Autodesk Fusion 360 part; units mm, degrees
(part 14 of 15)
  spline S147 degree 5 poles (-30.1889, -115.7087) (-30.196, -115.7166) (-30.2152, -115.7376) (-30.2465, -115.7718) (-30.29, -115.819) (-30.3459, -115.8792) (-30.4072, -115.9446) (-30.4688, -116.0097) (-30.5308, -116.0746) (-30.593, -116.1393) (-30.6557, -116.2038) (-30.7186, -116.268) (-30.7819, -116.332) (-30.8455, -116.3958) (-30.9093, -116.4594) (-30.9736, -116.5228) (-31.0381, -116.5859) (-31.1029, -116.6489) (-31.168, -116.7116) (-31.2334, -116.7741) (-31.2991, -116.8364) (-31.365, -116.8985) (-31.4313, -116.9604) (-31.4979, -117.0221) (-31.5647, -117.0836) (-31.6318, -117.1449) (-31.6992, -117.206) (-31.7668, -117.2669) (-31.8347, -117.3276) (-31.9029, -117.3881) (-31.9713, -117.4484) (-32.04, -117.5086) (-32.109, -117.5685) (-32.1782, -117.6282) (-32.2477, -117.6877) (-32.3174, -117.7471) (-32.3874, -117.8062) (-32.4576, -117.8652) (-32.5281, -117.9239) (-32.5988, -117.9825) (-32.6697, -118.0409) (-32.7409, -118.0991) (-32.8124, -118.1571) (-32.8697, -118.2034) (-32.9128, -118.238) (-32.9416, -118.261) (-32.956, -118.2725) knots 0.405839 0.405839 0.405839 0.405839 0.405839 0.405839 0.414286 0.428571 0.442857 0.457143 0.471429 0.485714 0.5 0.514286 0.528571 0.542857 0.557143 0.571429 0.585714 0.6 0.614286 0.628571 0.642857 0.657143 0.671429 0.685714 0.7 0.714286 0.728571 0.742857 0.757143 0.771429 0.785714 0.8 0.814286 0.828571 0.842857 0.857143 0.871429 0.885714 0.9 0.914286 0.928571 0.942857 0.957143 0.971429 0.985714 1 1 1 1 1 1
  arc A147 (-34.117, -117.6386) -> (-32.956, -118.2725) centre (2.0032, -52.8695) ccw
  spline S148 degree 5 poles (-34.117, -117.6386) (-34.1151, -117.6203) (-34.1113, -117.5836) (-34.1054, -117.5286) (-34.0975, -117.4554) (-34.0873, -117.3639) (-34.0769, -117.2726) (-34.0661, -117.1813) (-34.0551, -117.0901) (-34.0437, -116.9991) (-34.0321, -116.9081) (-34.0202, -116.8173) (-34.0079, -116.7266) (-33.9954, -116.6359) (-33.9826, -116.5454) (-33.9695, -116.455) (-33.956, -116.3647) (-33.9423, -116.2745) (-33.9283, -116.1845) (-33.9139, -116.0945) (-33.8993, -116.0047) (-33.8843, -115.915) (-33.869, -115.8254) (-33.8534, -115.7359) (-33.8375, -115.6466) (-33.8212, -115.5574) (-33.8046, -115.4683) (-33.7877, -115.3793) (-33.7705, -115.2905) (-33.7529, -115.2018) (-33.735, -115.1133) (-33.7168, -115.0249) (-33.6982, -114.9366) (-33.6792, -114.8485) (-33.6599, -114.7605) (-33.6403, -114.6727) (-33.6203, -114.585) (-33.5999, -114.4975) (-33.5792, -114.4101) (-33.5581, -114.3229) (-33.5366, -114.2358) (-33.5147, -114.149) (-33.4943, -114.0693) (-33.4781, -114.0072) (-33.4662, -113.9624) (-33.4589, -113.9349) (-33.4562, -113.9247) knots -1 -1 -1 -1 -1 -1 -0.985714 -0.971429 -0.957143 -0.942857 -0.928571 -0.914286 -0.9 -0.885714 -0.871429 -0.857143 -0.842857 -0.828571 -0.814286 -0.8 -0.785714 -0.771429 -0.757143 -0.742857 -0.728571 -0.714286 -0.7 -0.685714 -0.671429 -0.657143 -0.642857 -0.628571 -0.614286 -0.6 -0.585714 -0.571429 -0.557143 -0.542857 -0.528571 -0.514286 -0.5 -0.485714 -0.471429 -0.457143 -0.442857 -0.428571 -0.414286 -0.405839 -0.405839 -0.405839 -0.405839 -0.405839 -0.405839
  arc A148 (-34.5898, -113.2521) -> (-33.4562, -113.9247) centre (2.0032, -52.8695) ccw
  spline S149 degree 5 poles (-34.5898, -113.2521) (-34.5974, -113.2594) (-34.618, -113.279) (-34.6517, -113.3108) (-34.6985, -113.3549) (-34.7586, -113.4109) (-34.8243, -113.4718) (-34.8904, -113.5323) (-34.9569, -113.5927) (-35.0236, -113.6527) (-35.0907, -113.7126) (-35.158, -113.7721) (-35.2257, -113.8315) (-35.2937, -113.8906) (-35.3619, -113.9494) (-35.4305, -114.008) (-35.4994, -114.0664) (-35.5685, -114.1246) (-35.6379, -114.1825) (-35.7076, -114.2402) (-35.7776, -114.2977) (-35.8478, -114.3549) (-35.9183, -114.412) (-35.9891, -114.4687) (-36.0601, -114.5253) (-36.1314, -114.5817) (-36.203, -114.6378) (-36.2748, -114.6937) (-36.3469, -114.7494) (-36.4192, -114.8049) (-36.4918, -114.8602) (-36.5646, -114.9152) (-36.6377, -114.9701) (-36.711, -115.0247) (-36.7845, -115.0791) (-36.8583, -115.1334) (-36.9323, -115.1874) (-37.0065, -115.2412) (-37.081, -115.2947) (-37.1557, -115.3481) (-37.2307, -115.4013) (-37.3058, -115.4543) (-37.3812, -115.5071) (-37.4417, -115.5491) (-37.4872, -115.5806) (-37.5175, -115.6015) (-37.5327, -115.6119) knots 0.405839 0.405839 0.405839 0.405839 0.405839 0.405839 0.414286 0.428571 0.442857 0.457143 0.471429 0.485714 0.5 0.514286 0.528571 0.542857 0.557143 0.571429 0.585714 0.6 0.614286 0.628571 0.642857 0.657143 0.671429 0.685714 0.7 0.714286 0.728571 0.742857 0.757143 0.771429 0.785714 0.8 0.814286 0.828571 0.842857 0.857143 0.871429 0.885714 0.9 0.914286 0.928571 0.942857 0.957143 0.971429 0.985714 1 1 1 1 1 1
  arc A149 (-38.6455, -114.8968) -> (-37.5327, -115.6119) centre (2.0032, -52.8695) ccw
  spline S150 degree 5 poles (-38.6455, -114.8968) (-38.6423, -114.8786) (-38.6359, -114.8423) (-38.6262, -114.7879) (-38.613, -114.7154) (-38.5964, -114.6249) (-38.5794, -114.5345) (-38.5622, -114.4443) (-38.5446, -114.3541) (-38.5268, -114.2641) (-38.5087, -114.1742) (-38.4904, -114.0845) (-38.4717, -113.9949) (-38.4527, -113.9054) (-38.4335, -113.816) (-38.414, -113.7267) (-38.3941, -113.6376) (-38.374, -113.5487) (-38.3536, -113.4598) (-38.3328, -113.3711) (-38.3118, -113.2826) (-38.2905, -113.1942) (-38.2688, -113.1059) (-38.2469, -113.0178) (-38.2246, -112.9298) (-38.202, -112.842) (-38.1791, -112.7543) (-38.1559, -112.6668) (-38.1324, -112.5794) (-38.1086, -112.4922) (-38.0844, -112.4051) (-38.0599, -112.3183) (-38.035, -112.2316) (-38.0098, -112.145) (-37.9843, -112.0586) (-37.9584, -111.9724) (-37.9322, -111.8864) (-37.9057, -111.8005) (-37.8788, -111.7149) (-37.8515, -111.6294) (-37.8238, -111.5441) (-37.7958, -111.459) (-37.7698, -111.381) (-37.7492, -111.3202) (-37.7342, -111.2763) (-37.7249, -111.2494) (-37.7214, -111.2395) knots -1 -1 -1 -1 -1 -1 -0.985714 -0.971429 -0.957143 -0.942857 -0.928571 -0.914286 -0.9 -0.885714 -0.871429 -0.857143 -0.842857 -0.828571 -0.814286 -0.8 -0.785714 -0.771429 -0.757143 -0.742857 -0.728571 -0.714286 -0.7 -0.685714 -0.671429 -0.657143 -0.642857 -0.628571 -0.614286 -0.6 -0.585714 -0.571429 -0.557143 -0.542857 -0.528571 -0.514286 -0.5 -0.485714 -0.471429 -0.457143 -0.442857 -0.428571 -0.414286 -0.405839 -0.405839 -0.405839 -0.405839 -0.405839 -0.405839
  arc A150 (-38.8042, -110.4877) -> (-37.7214, -111.2395) centre (2.0032, -52.8695) ccw
  spline S151 degree 5 poles (-38.8042, -110.4877) (-38.8123, -110.4944) (-38.8343, -110.5125) (-38.8701, -110.5419) (-38.9199, -110.5825) (-38.9839, -110.6341) (-39.0538, -110.6901) (-39.1241, -110.7458) (-39.1946, -110.8012) (-39.2655, -110.8564) (-39.3367, -110.9113) (-39.4081, -110.9659) (-39.4798, -111.0203) (-39.5518, -111.0744) (-39.6241, -111.1282) (-39.6967, -111.1818) (-39.7695, -111.2351) (-39.8426, -111.2882) (-39.916, -111.341) (-39.9896, -111.3936) (-40.0635, -111.4459) (-40.1377, -111.498) (-40.2121, -111.5499) (-40.2867, -111.6015) (-40.3616, -111.6528) (-40.4368, -111.7039) (-40.5122, -111.7548) (-40.5878, -111.8055) (-40.6636, -111.8559) (-40.7397, -111.9061) (-40.8161, -111.956) (-40.8926, -112.0058) (-40.9694, -112.0553) (-41.0464, -112.1045) (-41.1237, -112.1536) (-41.2011, -112.2024) (-41.2788, -112.251) (-41.3567, -112.2993) (-41.4348, -112.3475) (-41.5131, -112.3954) (-41.5917, -112.4431) (-41.6704, -112.4906) (-41.7494, -112.5378) (-41.8127, -112.5754) (-41.8603, -112.6036) (-41.8921, -112.6223) (-41.908, -112.6316) knots 0.405839 0.405839 0.405839 0.405839 0.405839 0.405839 0.414286 0.428571 0.442857 0.457143 0.471429 0.485714 0.5 0.514286 0.528571 0.542857 0.557143 0.571429 0.585714 0.6 0.614286 0.628571 0.642857 0.657143 0.671429 0.685714 0.7 0.714286 0.728571 0.742857 0.757143 0.771429 0.785714 0.8 0.814286 0.828571 0.842857 0.857143 0.871429 0.885714 0.9 0.914286 0.928571 0.942857 0.957143 0.971429 0.985714 1 1 1 1 1 1
  arc A151 (-42.9669, -111.8389) -> (-41.908, -112.6316) centre (2.0032, -52.8695) ccw
  spline S152 degree 5 poles (-42.9669, -111.8389) (-42.9624, -111.821) (-42.9534, -111.7853) (-42.9399, -111.7317) (-42.9216, -111.6603) (-42.8985, -111.5712) (-42.8751, -111.4823) (-42.8515, -111.3935) (-42.8276, -111.3048) (-42.8034, -111.2163) (-42.7789, -111.128) (-42.7542, -111.0397) (-42.7292, -110.9517) (-42.7039, -110.8637) (-42.6783, -110.776) (-42.6525, -110.6884) (-42.6263, -110.6009) (-42.5999, -110.5136) (-42.5732, -110.4264) (-42.5462, -110.3394) (-42.5189, -110.2526) (-42.4913, -110.1659) (-42.4634, -110.0794) (-42.4353, -109.9931) (-42.4068, -109.9069) (-42.378, -109.8209) (-42.3489, -109.7351) (-42.3195, -109.6495) (-42.2898, -109.564) (-42.2598, -109.4787) (-42.2295, -109.3936) (-42.1988, -109.3087) (-42.1678, -109.224) (-42.1365, -109.1395) (-42.1049, -109.0551) (-42.073, -108.971) (-42.0407, -108.8871) (-42.0081, -108.8033) (-41.9751, -108.7198) (-41.9418, -108.6365) (-41.9082, -108.5534) (-41.8742, -108.4705) (-41.8426, -108.3946) (-41.8177, -108.3354) (-41.7996, -108.2927) (-41.7885, -108.2665) (-41.7843, -108.2568) knots -1 -1 -1 -1 -1 -1 -0.985714 -0.971429 -0.957143 -0.942857 -0.928571 -0.914286 -0.9 -0.885714 -0.871429 -0.857143 -0.842857 -0.828571 -0.814286 -0.8 -0.785714 -0.771429 -0.757143 -0.742857 -0.728571 -0.714286 -0.7 -0.685714 -0.671429 -0.657143 -0.642857 -0.628571 -0.614286 -0.6 -0.585714 -0.571429 -0.557143 -0.542857 -0.528571 -0.514286 -0.5 -0.485714 -0.471429 -0.457143 -0.442857 -0.428571 -0.414286 -0.405839 -0.405839 -0.405839 -0.405839 -0.405839 -0.405839
  arc A152 (-42.8106, -107.4297) -> (-41.7843, -108.2568) centre (2.0032, -52.8695) ccw
  spline S153 degree 5 poles (-42.8106, -107.4297) (-42.8193, -107.4359) (-42.8425, -107.4523) (-42.8803, -107.4791) (-42.9329, -107.516) (-43.0003, -107.563) (-43.0741, -107.6138) (-43.1481, -107.6644) (-43.2225, -107.7146) (-43.2971, -107.7646) (-43.372, -107.8142) (-43.4471, -107.8636) (-43.5226, -107.9127) (-43.5983, -107.9616) (-43.6742, -108.0101) (-43.7504, -108.0584) (-43.8269, -108.1064) (-43.9036, -108.1541) (-43.9805, -108.2016) (-44.0577, -108.2487) (-44.1352, -108.2957) (-44.2128, -108.3423) (-44.2907, -108.3887) (-44.3689, -108.4349) (-44.4472, -108.4808) (-44.5258, -108.5264) (-44.6047, -108.5718) (-44.6837, -108.6169) (-44.763, -108.6618) (-44.8425, -108.7064) (-44.9222, -108.7508) (-45.0021, -108.7949) (-45.0822, -108.8388) (-45.1625, -108.8825) (-45.2431, -108.9259) (-45.3238, -108.969) (-45.4047, -109.012) (-45.4859, -109.0546) (-45.5672, -109.0971) (-45.6488, -109.1393) (-45.7305, -109.1813) (-45.8125, -109.223) (-45.8946, -109.2645) (-45.9605, -109.2975) (-46.0099, -109.3222) (-46.043, -109.3386) (-46.0595, -109.3468) knots 0.405839 0.405839 0.405839 0.405839 0.405839 0.405839 0.414286 0.428571 0.442857 0.457143 0.471429 0.485714 0.5 0.514286 0.528571 0.542857 0.557143 0.571429 0.585714 0.6 0.614286 0.628571 0.642857 0.657143 0.671429 0.685714 0.7 0.714286 0.728571 0.742857 0.757143 0.771429 0.785714 0.8 0.814286 0.828571 0.842857 0.857143 0.871429 0.885714 0.9 0.914286 0.928571 0.942857 0.957143 0.971429 0.985714 1 1 1 1 1 1
  arc A153 (-47.0592, -108.4805) -> (-46.0595, -109.3468) centre (2.0032, -52.8695) ccw
  spline S154 degree 5 poles (-47.0592, -108.4805) (-47.0534, -108.463) (-47.0419, -108.428) (-47.0245, -108.3755) (-47.0012, -108.3056) (-46.9718, -108.2184) (-46.9422, -108.1314) (-46.9123, -108.0445) (-46.8821, -107.9578) (-46.8517, -107.8712) (-46.821, -107.7848) (-46.79, -107.6986) (-46.7588, -107.6125) (-46.7273, -107.5266) (-46.6955, -107.4409) (-46.6635, -107.3553) (-46.6311, -107.27) (-46.5986, -107.1848) (-46.5657, -107.0997) (-46.5326, -107.0149) (-46.4991, -106.9302) (-46.4654, -106.8457) (-46.4314, -106.7615) (-46.3972, -106.6774) (-46.3626, -106.5934) (-46.3278, -106.5097) (-46.2926, -106.4262) (-46.2572, -106.3429) (-46.2215, -106.2597) (-46.1855, -106.1768) (-46.1491, -106.0941) (-46.1125, -106.0116) (-46.0756, -105.9293) (-46.0383, -105.8472) (-46.0008, -105.7653) (-45.9629, -105.6837) (-45.9247, -105.6023) (-45.8862, -105.5211) (-45.8474, -105.4401) (-45.8082, -105.3594) (-45.7687, -105.2789) (-45.7289, -105.1987) (-45.692, -105.1252) (-45.663, -105.0679) (-45.6419, -105.0266) (-45.6289, -105.0013) (-45.624, -104.9919) knots -1 -1 -1 -1 -1 -1 -0.985714 -0.971429 -0.957143 -0.942857 -0.928571 -0.914286 -0.9 -0.885714 -0.871429 -0.857143 -0.842857 -0.828571 -0.814286 -0.8 -0.785714 -0.771429 -0.757143 -0.742857 -0.728571 -0.714286 -0.7 -0.685714 -0.671429 -0.657143 -0.642857 -0.628571 -0.614286 -0.6 -0.585714 -0.571429 -0.557143 -0.542857 -0.528571 -0.514286 -0.5 -0.485714 -0.471429 -0.457143 -0.442857 -0.428571 -0.414286 -0.405839 -0.405839 -0.405839 -0.405839 -0.405839 -0.405839
  arc A154 (-46.5887, -104.0937) -> (-45.624, -104.9919) centre (2.0032, -52.8695) ccw
  spline S155 degree 5 poles (-46.5887, -104.0937) (-46.5978, -104.0992) (-46.6221, -104.114) (-46.6617, -104.138) (-46.7168, -104.1711) (-46.7875, -104.2131) (-46.8647, -104.2586) (-46.9421, -104.3037) (-47.0199, -104.3485) (-47.0978, -104.393) (-47.1761, -104.4372) (-47.2546, -104.4811) (-47.3333, -104.5247) (-47.4123, -104.568) (-47.4915, -104.611) (-47.571, -104.6537) (-47.6506, -104.6962) (-47.7306, -104.7383) (-47.8107, -104.7801) (-47.8911, -104.8217) (-47.9717, -104.863) (-48.0525, -104.904) (-48.1335, -104.9447) (-48.2147, -104.9852) (-48.2962, -105.0253) (-48.3778, -105.0653) (-48.4597, -105.1049) (-48.5417, -105.1443) (-48.624, -105.1834) (-48.7065, -105.2222) (-48.7891, -105.2608) (-48.872, -105.2991) (-48.955, -105.3372) (-49.0383, -105.375) (-49.1217, -105.4125) (-49.2053, -105.4498) (-49.2891, -105.4869) (-49.3731, -105.5236) (-49.4573, -105.5602) (-49.5416, -105.5965) (-49.6261, -105.6325) (-49.7109, -105.6683) (-49.7957, -105.7038) (-49.8638, -105.7321) (-49.9149, -105.7531) (-49.949, -105.7671) (-49.9661, -105.7741) knots 0.405839 0.405839 0.405839 0.405839 0.405839 0.405839 0.414286 0.428571 0.442857 0.457143 0.471429 0.485714 0.5 0.514286 0.528571 0.542857 0.557143 0.571429 0.585714 0.6 0.614286 0.628571 0.642857 0.657143 0.671429 0.685714 0.7 0.714286 0.728571 0.742857 0.757143 0.771429 0.785714 0.8 0.814286 0.828571 0.842857 0.857143 0.871429 0.885714 0.9 0.914286 0.928571 0.942857 0.957143 0.971429 0.985714 1 1 1 1 1 1
  arc A155 (-50.9014, -104.8388) -> (-49.9661, -105.7741) centre (2.0032, -52.8695) ccw
  spline S156 degree 5 poles (-50.9014, -104.8388) (-50.8944, -104.8217) (-50.8804, -104.7876) (-50.8594, -104.7365) (-50.8311, -104.6684) (-50.7956, -104.5835) (-50.7598, -104.4988) (-50.7238, -104.4143) (-50.6875, -104.33) (-50.651, -104.2458) (-50.6142, -104.1618) (-50.5771, -104.078) (-50.5398, -103.9944) (-50.5023, -103.911) (-50.4645, -103.8277) (-50.4264, -103.7447) (-50.3881, -103.6618) (-50.3495, -103.5792) (-50.3107, -103.4967) (-50.2716, -103.4144) (-50.2322, -103.3324) (-50.1926, -103.2505) (-50.1527, -103.1689) (-50.1125, -103.0874) (-50.072, -103.0062) (-50.0313, -102.9252) (-49.9903, -102.8444) (-49.949, -102.7638) (-49.9074, -102.6834) (-49.8656, -102.6033) (-49.8235, -102.5233) (-49.781, -102.4437) (-49.7383, -102.3642) (-49.6953, -102.285) (-49.652, -102.206) (-49.6084, -102.1273) (-49.5645, -102.0488) (-49.5203, -101.9705) (-49.4758, -101.8926) (-49.431, -101.8148) (-49.3859, -101.7374) (-49.3404, -101.6602) (-49.2984, -101.5895) (-49.2653, -101.5344) (-49.2413, -101.4948) (-49.2265, -101.4705) (-49.221, -101.4614) knots -1 -1 -1 -1 -1 -1 -0.985714 -0.971429 -0.957143 -0.942857 -0.928571 -0.914286 -0.9 -0.885714 -0.871429 -0.857143 -0.842857 -0.828571 -0.814286 -0.8 -0.785714 -0.771429 -0.757143 -0.742857 -0.728571 -0.714286 -0.7 -0.685714 -0.671429 -0.657143 -0.642857 -0.628571 -0.614286 -0.6 -0.585714 -0.571429 -0.557143 -0.542857 -0.528571 -0.514286 -0.5 -0.485714 -0.471429 -0.457143 -0.442857 -0.428571 -0.414286 -0.405839 -0.405839 -0.405839 -0.405839 -0.405839 -0.405839
  arc A156 (-50.1192, -100.4967) -> (-49.221, -101.4614) centre (2.0032, -52.8695) ccw
  spline S157 degree 5 poles (-50.1192, -100.4967) (-50.1286, -100.5016) (-50.1539, -100.5146) (-50.1952, -100.5356) (-50.2525, -100.5647) (-50.326, -100.6016) (-50.4062, -100.6414) (-50.4867, -100.6809) (-50.5674, -100.7201) (-50.6484, -100.7589) (-50.7296, -100.7974) (-50.811, -100.8356) (-50.8927, -100.8735) (-50.9745, -100.911) (-51.0566, -100.9483) (-51.1389, -100.9852) (-51.2214, -101.0218) (-51.3041, -101.0582) (-51.3871, -101.0942) (-51.4702, -101.1299) (-51.5535, -101.1653) (-51.637, -101.2005) (-51.7207, -101.2353) (-51.8047, -101.2699) (-51.8888, -101.3041) (-51.9731, -101.3381) (-52.0575, -101.3718) (-52.1422, -101.4052) (-52.227, -101.4384) (-52.3121, -101.4712) (-52.3973, -101.5038) (-52.4826, -101.5361) (-52.5682, -101.5682) (-52.6539, -101.6) (-52.7398, -101.6315) (-52.8259, -101.6627) (-52.9121, -101.6936) (-52.9985, -101.7243) (-53.0851, -101.7548) (-53.1718, -101.785) (-53.2587, -101.8149) (-53.3457, -101.8445) (-53.4329, -101.8739) (-53.5028, -101.8972) (-53.5553, -101.9146) (-53.5903, -101.9261) (-53.6078, -101.9319) knots 0.405839 0.405839 0.405839 0.405839 0.405839 0.405839 0.414286 0.428571 0.442857 0.457143 0.471429 0.485714 0.5 0.514286 0.528571 0.542857 0.557143 0.571429 0.585714 0.6 0.614286 0.628571 0.642857 0.657143 0.671429 0.685714 0.7 0.714286 0.728571 0.742857 0.757143 0.771429 0.785714 0.8 0.814286 0.828571 0.842857 0.857143 0.871429 0.885714 0.9 0.914286 0.928571 0.942857 0.957143 0.971429 0.985714 1 1 1 1 1 1
  arc A157 (-54.4741, -100.9322) -> (-53.6078, -101.9319) centre (2.0032, -52.8695) ccw
  spline S158 degree 5 poles (-54.4741, -100.9322) (-54.4659, -100.9157) (-54.4495, -100.8826) (-54.4248, -100.8331) (-54.3918, -100.7673) (-54.3503, -100.6852) (-54.3086, -100.6032) (-54.2666, -100.5215) (-54.2244, -100.4399) (-54.1819, -100.3586) (-54.1393, -100.2774) (-54.0963, -100.1965) (-54.0532, -100.1157) (-54.0098, -100.0352) (-53.9661, -99.9549) (-53.9222, -99.8748) (-53.8781, -99.7948) (-53.8337, -99.7152) (-53.7891, -99.6357) (-53.7442, -99.5564) (-53.6991, -99.4774) (-53.6537, -99.3985) (-53.6081, -99.3199) (-53.5622, -99.2416) (-53.516, -99.1634) (-53.4696, -99.0855) (-53.423, -99.0078) (-53.3761, -98.9304) (-53.3289, -98.8532) (-53.2814, -98.7763) (-53.2337, -98.6996) (-53.1857, -98.6231) (-53.1374, -98.5469) (-53.0889, -98.4709) (-53.04, -98.3953) (-52.9909, -98.3198) (-52.9416, -98.2447) (-52.8919, -98.1698) (-52.8419, -98.0952) (-52.7917, -98.0208) (-52.7411, -97.9468) (-52.6903, -97.873) (-52.6433, -97.8056) (-52.6064, -97.753) (-52.5796, -97.7151) (-52.5632, -97.6919) (-52.557, -97.6833) knots -1 -1 -1 -1 -1 -1 -0.985714 -0.971429 -0.957143 -0.942857 -0.928571 -0.914286 -0.9 -0.885714 -0.871429 -0.857143 -0.842857 -0.828571 -0.814286 -0.8 -0.785714 -0.771429 -0.757143 -0.742857 -0.728571 -0.714286 -0.7 -0.685714 -0.671429 -0.657143 -0.642857 -0.628571 -0.614286 -0.6 -0.585714 -0.571429 -0.557143 -0.542857 -0.528571 -0.514286 -0.5 -0.485714 -0.471429 -0.457143 -0.442857 -0.428571 -0.414286 -0.405839 -0.405839 -0.405839 -0.405839 -0.405839 -0.405839
  arc A158 (-53.3841, -96.657) -> (-52.557, -97.6833) centre (2.0032, -52.8695) ccw
  spline S159 degree 5 poles (-53.3841, -96.657) (-53.3938, -96.6611) (-53.42, -96.6723) (-53.4627, -96.6904) (-53.5219, -96.7153) (-53.5978, -96.7469) (-53.6807, -96.7809) (-53.7638, -96.8145) (-53.8471, -96.8478) (-53.9306, -96.8808) (-54.0144, -96.9134) (-54.0983, -96.9457) (-54.1824, -96.9776) (-54.2668, -97.0092) (-54.3513, -97.0405) (-54.436, -97.0715) (-54.5209, -97.1021) (-54.606, -97.1325) (-54.6913, -97.1625) (-54.7768, -97.1922) (-54.8624, -97.2216) (-54.9483, -97.2507) (-55.0342, -97.2795) (-55.1204, -97.3079) (-55.2067, -97.3361) (-55.2932, -97.364) (-55.3799, -97.3916) (-55.4667, -97.4189) (-55.5537, -97.4459) (-55.6409, -97.4726) (-55.7282, -97.499) (-55.8157, -97.5252) (-55.9033, -97.551) (-55.991, -97.5766) (-56.079, -97.6019) (-56.167, -97.6269) (-56.2553, -97.6516) (-56.3436, -97.6761) (-56.4321, -97.7003) (-56.5208, -97.7242) (-56.6096, -97.7478) (-56.6985, -97.7712) (-56.7876, -97.7943) (-56.859, -97.8126) (-56.9126, -97.8261) (-56.9483, -97.8351) (-56.9662, -97.8396) knots 0.405839 0.405839 0.405839 0.405839 0.405839 0.405839 0.414286 0.428571 0.442857 0.457143 0.471429 0.485714 0.5 0.514286 0.528571 0.542857 0.557143 0.571429 0.585714 0.6 0.614286 0.628571 0.642857 0.657143 0.671429 0.685714 0.7 0.714286 0.728571 0.742857 0.757143 0.771429 0.785714 0.8 0.814286 0.828571 0.842857 0.857143 0.871429 0.885714 0.9 0.914286 0.928571 0.942857 0.957143 0.971429 0.985714 1 1 1 1 1 1
  arc A159 (-57.7589, -96.7807) -> (-56.9662, -97.8396) centre (2.0032, -52.8695) ccw
  spline S160 degree 5 poles (-57.7589, -96.7807) (-57.7496, -96.7648) (-57.7309, -96.733) (-57.7027, -96.6854) (-57.6651, -96.6221) (-57.6179, -96.5431) (-57.5704, -96.4644) (-57.5227, -96.3858) (-57.4748, -96.3075) (-57.4266, -96.2294) (-57.3783, -96.1515) (-57.3297, -96.0738) (-57.2809, -95.9964) (-57.2318, -95.9191) (-57.1826, -95.8421) (-57.1331, -95.7653) (-57.0833, -95.6888) (-57.0334, -95.6124) (-56.9832, -95.5363) (-56.9328, -95.4605) (-56.8821, -95.3849) (-56.8313, -95.3095) (-56.7801, -95.2343) (-56.7288, -95.1594) (-56.6772, -95.0848) (-56.6253, -95.0104) (-56.5732, -94.9362) (-56.5209, -94.8623) (-56.4683, -94.7887) (-56.4155, -94.7153) (-56.3624, -94.6422) (-56.3091, -94.5694) (-56.2555, -94.4968) (-56.2017, -94.4245) (-56.1476, -94.3525) (-56.0932, -94.2808) (-56.0386, -94.2093) (-55.9837, -94.1382) (-55.9285, -94.0673) (-55.8731, -93.9968) (-55.8174, -93.9265) (-55.7614, -93.8566) (-55.7098, -93.7926) (-55.6692, -93.7428) (-55.6398, -93.707) (-55.6217, -93.685) (-55.615, -93.6769) knots -1 -1 -1 -1 -1 -1 -0.985714 -0.971429 -0.957143 -0.942857 -0.928571 -0.914286 -0.9 -0.885714 -0.871429 -0.857143 -0.842857 -0.828571 -0.814286 -0.8 -0.785714 -0.771429 -0.757143 -0.742857 -0.728571 -0.714286 -0.7 -0.685714 -0.671429 -0.657143 -0.642857 -0.628571 -0.614286 -0.6 -0.585714 -0.571429 -0.557143 -0.542857 -0.528571 -0.514286 -0.5 -0.485714 -0.471429 -0.457143 -0.442857 -0.428571 -0.414286 -0.405839 -0.405839 -0.405839 -0.405839 -0.405839 -0.405839
  arc A160 (-56.3668, -92.5941) -> (-55.615, -93.6769) centre (2.0032, -52.8695) ccw
  spline S161 degree 5 poles (-56.3668, -92.5941) (-56.3768, -92.5976) (-56.4037, -92.6069) (-56.4475, -92.6219) (-56.5083, -92.6425) (-56.5863, -92.6685) (-56.6714, -92.6965) (-56.7567, -92.7242) (-56.8422, -92.7515) (-56.9278, -92.7784) (-57.0137, -92.8049) (-57.0997, -92.8311) (-57.1859, -92.857) (-57.2723, -92.8825) (-57.3589, -92.9077) (-57.4456, -92.9325) (-57.5325, -92.9571) (-57.6195, -92.9812) (-57.7067, -93.0051) (-57.7941, -93.0286) (-57.8816, -93.0518) (-57.9693, -93.0747) (-58.0571, -93.0973) (-58.1451, -93.1196) (-58.2332, -93.1415) (-58.3215, -93.1632) (-58.4099, -93.1845) (-58.4984, -93.2055) (-58.5871, -93.2263) (-58.676, -93.2467) (-58.7649, -93.2668) (-58.854, -93.2866) (-58.9433, -93.3062) (-59.0327, -93.3254) (-59.1222, -93.3444) (-59.2118, -93.363) (-59.3016, -93.3814) (-59.3914, -93.3995) (-59.4815, -93.4173) (-59.5716, -93.4348) (-59.6618, -93.4521) (-59.7522, -93.4691) (-59.8427, -93.4857) (-59.9152, -93.4989) (-59.9696, -93.5086) (-60.0059, -93.515) (-60.0241, -93.5182) knots 0.405839 0.405839 0.405839 0.405839 0.405839 0.405839 0.414286 0.428571 0.442857 0.457143 0.471429 0.485714 0.5 0.514286 0.528571 0.542857 0.557143 0.571429 0.585714 0.6 0.614286 0.628571 0.642857 0.657143 0.671429 0.685714 0.7 0.714286 0.728571 0.742857 0.757143 0.771429 0.785714 0.8 0.814286 0.828571 0.842857 0.857143 0.871429 0.885714 0.9 0.914286 0.928571 0.942857 0.957143 0.971429 0.985714 1 1 1 1 1 1
  arc A161 (-60.7392, -92.4054) -> (-60.0241, -93.5182) centre (2.0032, -52.8695) ccw
  spline S162 degree 5 poles (-60.7392, -92.4054) (-60.7288, -92.3902) (-60.7079, -92.3599) (-60.6764, -92.3144) (-60.6344, -92.2539) (-60.5816, -92.1785) (-60.5286, -92.1034) (-60.4754, -92.0284) (-60.4221, -91.9537) (-60.3685, -91.8792) (-60.3147, -91.805) (-60.2607, -91.731) (-60.2065, -91.6572) (-60.152, -91.5837) (-60.0974, -91.5103) (-60.0426, -91.4373) (-59.9875, -91.3645) (-59.9322, -91.2919) (-59.8767, -91.2196) (-59.821, -91.1475) (-59.7651, -91.0757) (-59.709, -91.0041) (-59.6526, -90.9328) (-59.5961, -90.8618) (-59.5393, -90.791) (-59.4822, -90.7205) (-59.425, -90.6503) (-59.3675, -90.5803) (-59.3098, -90.5106) (-59.2519, -90.4412) (-59.1937, -90.372) (-59.1354, -90.3032) (-59.0767, -90.2346) (-59.0179, -90.1664) (-58.9588, -90.0984) (-58.8994, -90.0307) (-58.8399, -89.9634) (-58.78, -89.8963) (-58.72, -89.8296) (-58.6596, -89.7631) (-58.5991, -89.697) (-58.5383, -89.6313) (-58.4822, -89.5712) (-58.4381, -89.5244) (-58.4063, -89.4907) (-58.3867, -89.4701) (-58.3794, -89.4625) knots -1 -1 -1 -1 -1 -1 -0.985714 -0.971429 -0.957143 -0.942857 -0.928571 -0.914286 -0.9 -0.885714 -0.871429 -0.857143 -0.842857 -0.828571 -0.814286 -0.8 -0.785714 -0.771429 -0.757143 -0.742857 -0.728571 -0.714286 -0.7 -0.685714 -0.671429 -0.657143 -0.642857 -0.628571 -0.614286 -0.6 -0.585714 -0.571429 -0.557143 -0.542857 -0.528571 -0.514286 -0.5 -0.485714 -0.471429 -0.457143 -0.442857 -0.428571 -0.414286 -0.405839 -0.405839 -0.405839 -0.405839 -0.405839 -0.405839
  arc A162 (-59.052, -88.3289) -> (-58.3794, -89.4625) centre (2.0032, -52.8695) ccw
  spline S163 degree 5 poles (-59.052, -88.3289) (-59.0622, -88.3316) (-59.0897, -88.3389) (-59.1345, -88.3508) (-59.1966, -88.367) (-59.2763, -88.3874) (-59.3631, -88.4093) (-59.4502, -88.4307) (-59.5374, -88.4519) (-59.6248, -88.4726) (-59.7123, -88.493) (-59.8, -88.513) (-59.8878, -88.5326) (-59.9758, -88.5519) (-60.0639, -88.5709) (-60.1522, -88.5894) (-60.2406, -88.6077) (-60.3291, -88.6256) (-60.4178, -88.6432) (-60.5066, -88.6604) (-60.5956, -88.6773) (-60.6847, -88.6939) (-60.7739, -88.7102) (-60.8632, -88.7261) (-60.9527, -88.7417) (-61.0423, -88.757) (-61.132, -88.772) (-61.2218, -88.7866) (-61.3118, -88.801) (-61.4018, -88.815) (-61.492, -88.8287) (-61.5823, -88.8422) (-61.6727, -88.8553) (-61.7632, -88.8681) (-61.8539, -88.8806) (-61.9446, -88.8928) (-62.0354, -88.9048) (-62.1264, -88.9164) (-62.2174, -88.9277) (-62.3086, -88.9388) (-62.3999, -88.9496) (-62.4912, -88.96) (-62.5827, -88.9702) (-62.6559, -88.9781) (-62.7109, -88.9839) (-62.7476, -88.9878) (-62.7659, -88.9897) knots 0.405839 0.405839 0.405839 0.405839 0.405839 0.405839 0.414286 0.428571 0.442857 0.457143 0.471429 0.485714 0.5 0.514286 0.528571 0.542857 0.557143 0.571429 0.585714 0.6 0.614286 0.628571 0.642857 0.657143 0.671429 0.685714 0.7 0.714286 0.728571 0.742857 0.757143 0.771429 0.785714 0.8 0.814286 0.828571 0.842857 0.857143 0.871429 0.885714 0.9 0.914286 0.928571 0.942857 0.957143 0.971429 0.985714 1 1 1 1 1 1
  arc A163 (-63.3998, -87.8287) -> (-62.7659, -88.9897) centre (2.0032, -52.8695) ccw
  spline S164 degree 5 poles (-63.3998, -87.8287) (-63.3883, -87.8143) (-63.3653, -87.7855) (-63.3307, -87.7424) (-63.2844, -87.6851) (-63.2264, -87.6136) (-63.1682, -87.5424) (-63.1098, -87.4715) (-63.0512, -87.4008) (-62.9925, -87.3303) (-62.9335, -87.2601) (-62.8744, -87.1901) (-62.815, -87.1204) (-62.7555, -87.0509) (-62.6958, -86.9817) (-62.6359, -86.9127) (-62.5757, -86.844) (-62.5154, -86.7756) (-62.4549, -86.7074) (-62.3942, -86.6395) (-62.3333, -86.5718) (-62.2722, -86.5045) (-62.2109, -86.4374) (-62.1494, -86.3705) (-62.0877, -86.304) (-62.0258, -86.2377) (-61.9637, -86.1718) (-61.9014, -86.1061) (-61.8389, -86.0407) (-61.7762, -85.9756) (-61.7132, -85.9108) (-61.6501, -85.8462) (-61.5867, -85.782) (-61.5231, -85.7181) (-61.4593, -85.6546) (-61.3953, -85.5913) (-61.3311, -85.5284) (-61.2666, -85.4657) (-61.202, -85.4035) (-61.137, -85.3415) (-61.0719, -85.2799) (-61.0066, -85.2186) (-60.9463, -85.1627) (-60.8991, -85.1191) (-60.8649, -85.0879) (-60.8439, -85.0687) (-60.836, -85.0616) knots -1 -1 -1 -1 -1 -1 -0.985714 -0.971429 -0.957143 -0.942857 -0.928571 -0.914286 -0.9 -0.885714 -0.871429 -0.857143 -0.842857 -0.828571 -0.814286 -0.8 -0.785714 -0.771429 -0.757143 -0.742857 -0.728571 -0.714286 -0.7 -0.685714 -0.671429 -0.657143 -0.642857 -0.628571 -0.614286 -0.6 -0.585714 -0.571429 -0.557143 -0.542857 -0.528571 -0.514286 -0.5 -0.485714 -0.471429 -0.457143 -0.442857 -0.428571 -0.414286 -0.405839 -0.405839 -0.405839 -0.405839 -0.405839 -0.405839
  arc A164 (-61.4261, -83.8829) -> (-60.836, -85.0616) centre (2.0032, -52.8695) ccw
  spline S165 degree 5 poles (-61.4261, -83.8829) (-61.4364, -83.8849) (-61.4644, -83.8902) (-61.5099, -83.8988) (-61.5731, -83.9106) (-61.654, -83.9253) (-61.7422, -83.9409) (-61.8305, -83.9561) (-61.919, -83.9709) (-62.0076, -83.9854) (-62.0964, -83.9995) (-62.1853, -84.0132) (-62.2743, -84.0265) (-62.3634, -84.0395) (-62.4527, -84.0521) (-62.542, -84.0643) (-62.6315, -84.0762) (-62.7211, -84.0878) (-62.8108, -84.099) (-62.9007, -84.1098) (-62.9906, -84.1203) (-63.0806, -84.1305) (-63.1708, -84.1404) (-63.261, -84.1499) (-63.3514, -84.1591) (-63.4418, -84.1679) (-63.5324, -84.1765) (-63.623, -84.1847) (-63.7138, -84.1926) (-63.8046, -84.2002) (-63.8955, -84.2074) (-63.9866, -84.2144) (-64.0777, -84.221) (-64.1689, -84.2273) (-64.2602, -84.2334) (-64.3515, -84.2391) (-64.443, -84.2445) (-64.5346, -84.2496) (-64.6262, -84.2544) (-64.7179, -84.2589) (-64.8097, -84.2632) (-64.9016, -84.2671) (-64.9935, -84.2707) (-65.0671, -84.2734) (-65.1224, -84.2753) (-65.1592, -84.2765) (-65.1777, -84.2771) knots 0.405839 0.405839 0.405839 0.405839 0.405839 0.405839 0.414286 0.428571 0.442857 0.457143 0.471429 0.485714 0.5 0.514286 0.528571 0.542857 0.557143 0.571429 0.585714 0.6 0.614286 0.628571 0.642857 0.657143 0.671429 0.685714 0.7 0.714286 0.728571 0.742857 0.757143 0.771429 0.785714 0.8 0.814286 0.828571 0.842857 0.857143 0.871429 0.885714 0.9 0.914286 0.928571 0.942857 0.957143 0.971429 0.985714 1 1 1 1 1 1
  arc A165 (-65.7272, -83.0738) -> (-65.1777, -84.2771) centre (2.0032, -52.8695) ccw
  spline S166 degree 5 poles (-65.7272, -83.0738) (-65.7147, -83.0603) (-65.6896, -83.0332) (-65.652, -82.9927) (-65.6018, -82.9388) (-65.5388, -82.8717) (-65.4757, -82.8048) (-65.4124, -82.7382) (-65.3489, -82.6719) (-65.2853, -82.6058) (-65.2215, -82.5399) (-65.1575, -82.4743) (-65.0933, -82.409) (-65.029, -82.344) (-64.9645, -82.2792) (-64.8998, -82.2147) (-64.8349, -82.1505) (-64.7699, -82.0865) (-64.7047, -82.0228) (-64.6393, -81.9594) (-64.5737, -81.8963) (-64.508, -81.8334) (-64.442, -81.7709) (-64.3759, -81.7086) (-64.3096, -81.6466) (-64.2432, -81.5849) (-64.1765, -81.5236) (-64.1097, -81.4625) (-64.0426, -81.4017) (-63.9754, -81.3412) (-63.908, -81.2811) (-63.8404, -81.2213) (-63.7726, -81.1617) (-63.7047, -81.1025) (-63.6365, -81.0437) (-63.5681, -80.9851) (-63.4996, -80.9269) (-63.4308, -80.8691) (-63.3619, -80.8116) (-63.2927, -80.7544) (-63.2233, -80.6976) (-63.1538, -80.6411) (-63.0897, -80.5896) (-63.0395, -80.5496) (-63.0031, -80.5208) (-62.9808, -80.5032) (-62.9725, -80.4967) knots -1 -1 -1 -1 -1 -1 -0.985714 -0.971429 -0.957143 -0.942857 -0.928571 -0.914286 -0.9 -0.885714 -0.871429 -0.857143 -0.842857 -0.828571 -0.814286 -0.8 -0.785714 -0.771429 -0.757143 -0.742857 -0.728571 -0.714286 -0.7 -0.685714 -0.671429 -0.657143 -0.642857 -0.628571 -0.614286 -0.6 -0.585714 -0.571429 -0.557143 -0.542857 -0.528571 -0.514286 -0.5 -0.485714 -0.471429 -0.457143 -0.442857 -0.428571 -0.414286 -0.405839 -0.405839 -0.405839 -0.405839 -0.405839 -0.405839
  arc A166 (-63.4769, -79.2789) -> (-62.9725, -80.4967) centre (2.0032, -52.8695) ccw
  spline S167 degree 5 poles (-63.4769, -79.2789) (-63.4874, -79.2801) (-63.5157, -79.2835) (-63.5617, -79.2888) (-63.6255, -79.296) (-63.7073, -79.3049) (-63.7964, -79.3142) (-63.8856, -79.3231) (-63.9749, -79.3315) (-64.0643, -79.3396) (-64.1539, -79.3473) (-64.2435, -79.3547) (-64.3332, -79.3616) (-64.4231, -79.3682) (-64.513, -79.3744) (-64.603, -79.3802) (-64.6931, -79.3857) (-64.7833, -79.3908) (-64.8736, -79.3956) (-64.964, -79.4) (-65.0544, -79.4041) (-65.1449, -79.4078) (-65.2356, -79.4112) (-65.3263, -79.4143) (-65.417, -79.417) (-65.5079, -79.4194) (-65.5988, -79.4214) (-65.6898, -79.4232) (-65.7809, -79.4246) (-65.872, -79.4257) (-65.9633, -79.4264) (-66.0545, -79.4268) (-66.1459, -79.427) (-66.2373, -79.4268) (-66.3288, -79.4263) (-66.4204, -79.4255) (-66.512, -79.4243) (-66.6037, -79.4229) (-66.6954, -79.4212) (-66.7872, -79.4191) (-66.8791, -79.4168) (-66.971, -79.4142) (-67.0629, -79.4112) (-67.1366, -79.4086) (-67.1918, -79.4066) (-67.2287, -79.4051) (-67.2471, -79.4044) knots 0.405839 0.405839 0.405839 0.405839 0.405839 0.405839 0.414286 0.428571 0.442857 0.457143 0.471429 0.485714 0.5 0.514286 0.528571 0.542857 0.557143 0.571429 0.585714 0.6 0.614286 0.628571 0.642857 0.657143 0.671429 0.685714 0.7 0.714286 0.728571 0.742857 0.757143 0.771429 0.785714 0.8 0.814286 0.828571 0.842857 0.857143 0.871429 0.885714 0.9 0.914286 0.928571 0.942857 0.957143 0.971429 0.985714 1 1 1 1 1 1
  arc A167 (-67.7093, -78.165) -> (-67.2471, -79.4044) centre (2.0032, -52.8695) ccw
  spline S168 degree 5 poles (-67.7093, -78.165) (-67.6959, -78.1524) (-67.669, -78.1272) (-67.6286, -78.0894) (-67.5747, -78.0393) (-67.5071, -77.9768) (-67.4393, -77.9146) (-67.3714, -77.8527) (-67.3034, -77.7911) (-67.2352, -77.7297) (-67.1668, -77.6686) (-67.0983, -77.6077) (-67.0297, -77.5472) (-66.9609, -77.4869) (-66.8919, -77.4269) (-66.8228, -77.3671) (-66.7535, -77.3077) (-66.6841, -77.2485) (-66.6145, -77.1896) (-66.5447, -77.131) (-66.4748, -77.0728) (-66.4048, -77.0148) (-66.3345, -76.9571) (-66.2642, -76.8997) (-66.1936, -76.8426) (-66.1229, -76.7858) (-66.052, -76.7293) (-65.981, -76.6732) (-65.9098, -76.6174) (-65.8385, -76.5618) (-65.7669, -76.5066) (-65.6953, -76.4518) (-65.6234, -76.3973) (-65.5514, -76.3431) (-65.4792, -76.2892) (-65.4068, -76.2357) (-65.3343, -76.1825) (-65.2616, -76.1297) (-65.1887, -76.0773) (-65.1156, -76.0252) (-65.0424, -75.9735) (-64.969, -75.9221) (-64.9014, -75.8753) (-64.8484, -75.839) (-64.8101, -75.8129) (-64.7866, -75.7969) (-64.7778, -75.791) knots -1 -1 -1 -1 -1 -1 -0.985714 -0.971429 -0.957143 -0.942857 -0.928571 -0.914286 -0.9 -0.885714 -0.871429 -0.857143 -0.842857 -0.828571 -0.814286 -0.8 -0.785714 -0.771429 -0.757143 -0.742857 -0.728571 -0.714286 -0.7 -0.685714 -0.671429 -0.657143 -0.642857 -0.628571 -0.614286 -0.6 -0.585714 -0.571429 -0.557143 -0.542857 -0.528571 -0.514286 -0.5 -0.485714 -0.471429 -0.457143 -0.442857 -0.428571 -0.414286 -0.405839 -0.405839 -0.405839 -0.405839 -0.405839 -0.405839
  arc A168 (-65.1941, -74.5403) -> (-64.7778, -75.791) centre (2.0032, -52.8695) ccw
  spline S169 degree 5 poles (-65.1941, -74.5403) (-65.2047, -74.5408) (-65.2331, -74.5421) (-65.2794, -74.5441) (-65.3436, -74.5468) (-65.4257, -74.5498) (-65.5153, -74.5527) (-65.6049, -74.5552) (-65.6946, -74.5573) (-65.7844, -74.559) (-65.8742, -74.5603) (-65.9641, -74.5612) (-66.0541, -74.5617) (-66.1442, -74.5619) (-66.2343, -74.5616) (-66.3246, -74.5611) (-66.4148, -74.5601) (-66.5052, -74.5588) (-66.5955, -74.5571) (-66.686, -74.5551) (-66.7765, -74.5527) (-66.8671, -74.5499) (-66.9577, -74.5469) (-67.0484, -74.5434) (-67.1391, -74.5397) (-67.2299, -74.5356) (-67.3208, -74.5311) (-67.4117, -74.5264) (-67.5026, -74.5213) (-67.5936, -74.5158) (-67.6846, -74.5101) (-67.7757, -74.504) (-67.8669, -74.4976) (-67.958, -74.4909) (-68.0493, -74.4839) (-68.1405, -74.4765) (-68.2318, -74.4689) (-68.3232, -74.4609) (-68.4145, -74.4526) (-68.506, -74.444) (-68.5974, -74.4352) (-68.6889, -74.426) (-68.7804, -74.4165) (-68.8537, -74.4087) (-68.9087, -74.4026) (-68.9453, -74.3986) (-68.9636, -74.3965) knots 0.405839 0.405839 0.405839 0.405839 0.405839 0.405839 0.414286 0.428571 0.442857 0.457143 0.471429 0.485714 0.5 0.514286 0.528571 0.542857 0.557143 0.571429 0.585714 0.6 0.614286 0.628571 0.642857 0.657143 0.671429 0.685714 0.7 0.714286 0.728571 0.742857 0.757143 0.771429 0.785714 0.8 0.814286 0.828571 0.842857 0.857143 0.871429 0.885714 0.9 0.914286 0.928571 0.942857 0.957143 0.971429 0.985714 1 1 1 1 1 1
  arc A169 (-69.3363, -73.1273) -> (-68.9636, -74.3965) centre (2.0032, -52.8695) ccw
  spline S170 degree 5 poles (-69.3363, -73.1273) (-69.322, -73.1157) (-69.2934, -73.0925) (-69.2504, -73.0577) (-69.193, -73.0115) (-69.1211, -72.9541) (-69.0491, -72.8969) (-68.977, -72.8399) (-68.9047, -72.7833) (-68.8323, -72.7269) (-68.7598, -72.6709) (-68.6871, -72.615) (-68.6143, -72.5595) (-68.5413, -72.5043) (-68.4683, -72.4494) (-68.3951, -72.3947) (-68.3217, -72.3404) (-68.2482, -72.2863) (-68.1746, -72.2325) (-68.1009, -72.1791) (-68.027, -72.1259) (-67.953, -72.0731) (-67.8788, -72.0205) (-67.8045, -71.9683) (-67.7301, -71.9164) (-67.6555, -71.8648) (-67.5808, -71.8135) (-67.5059, -71.7626) (-67.4309, -71.712) (-67.3558, -71.6617) (-67.2805, -71.6118) (-67.2051, -71.5621) (-67.1295, -71.5129) (-67.0538, -71.464) (-66.978, -71.4154) (-66.902, -71.3672) (-66.8258, -71.3193) (-66.7496, -71.2718) (-66.6731, -71.2247) (-66.5965, -71.178) (-66.5198, -71.1316) (-66.4429, -71.0856) (-66.3721, -71.0438) (-66.3167, -71.0113) (-66.2767, -70.988) (-66.252, -70.9737) (-66.2429, -70.9684) knots -1 -1 -1 -1 -1 -1 -0.985714 -0.971429 -0.957143 -0.942857 -0.928571 -0.914286 -0.9 -0.885714 -0.871429 -0.857143 -0.842857 -0.828571 -0.814286 -0.8 -0.785714 -0.771429 -0.757143 -0.742857 -0.728571 -0.714286 -0.7 -0.685714 -0.671429 -0.657143 -0.642857 -0.628571 -0.614286 -0.6 -0.585714 -0.571429 -0.557143 -0.542857 -0.528571 -0.514286 -0.5 -0.485714 -0.471429 -0.457143 -0.442857 -0.428571 -0.414286 -0.405839 -0.405839 -0.405839 -0.405839 -0.405839 -0.405839
  arc A170 (-66.5689, -69.6913) -> (-66.2429, -70.9684) centre (2.0032, -52.8695) ccw
  spline S171 degree 5 poles (-66.5689, -69.6913) (-66.5794, -69.691) (-66.6079, -69.6903) (-66.6542, -69.689) (-66.7184, -69.6871) (-66.8006, -69.6843) (-66.8901, -69.6808) (-66.9797, -69.6768) (-67.0693, -69.6725) (-67.159, -69.6678) (-67.2487, -69.6627) (-67.3384, -69.6572) (-67.4282, -69.6513) (-67.5181, -69.645) (-67.608, -69.6384) (-67.6979, -69.6313) (-67.7879, -69.6239) (-67.8779, -69.6162) (-67.9679, -69.6081) (-68.058, -69.5996) (-68.1481, -69.5907) (-68.2383, -69.5815) (-68.3285, -69.572) (-68.4187, -69.5621) (-68.5089, -69.5519) (-68.5992, -69.5413) (-68.6895, -69.5304) (-68.7798, -69.5192) (-68.8701, -69.5076) (-68.9605, -69.4957) (-69.0509, -69.4835) (-69.1413, -69.4709) (-69.2318, -69.458) (-69.3222, -69.4448) (-69.4127, -69.4313) (-69.5032, -69.4175) (-69.5937, -69.4033) (-69.6843, -69.3889) (-69.7748, -69.3741) (-69.8654, -69.359) (-69.956, -69.3436) (-70.0466, -69.3279) (-70.1372, -69.3119) (-70.2097, -69.2989) (-70.2641, -69.289) (-70.3004, -69.2823) (-70.3185, -69.279) knots 0.405839 0.405839 0.405839 0.405839 0.405839 0.405839 0.414286 0.428571 0.442857 0.457143 0.471429 0.485714 0.5 0.514286 0.528571 0.542857 0.557143 0.571429 0.585714 0.6 0.614286 0.628571 0.642857 0.657143 0.671429 0.685714 0.7 0.714286 0.728571 0.742857 0.757143 0.771429 0.785714 0.8 0.814286 0.828571 0.842857 0.857143 0.871429 0.885714 0.9 0.914286 0.928571 0.942857 0.957143 0.971429 0.985714 1 1 1 1 1 1
  arc A171 (-70.5997, -67.9864) -> (-70.3185, -69.279) centre (2.0032, -52.8695) ccw
  spline S172 degree 5 poles (-70.5997, -67.9864) (-70.5846, -67.9758) (-70.5544, -67.9547) (-70.509, -67.9231) (-70.4485, -67.8811) (-70.3727, -67.8289) (-70.2968, -67.777) (-70.2208, -67.7254) (-70.1447, -67.6741) (-70.0684, -67.623) (-69.9921, -67.5722) (-69.9156, -67.5218) (-69.839, -67.4716) (-69.7623, -67.4217) (-69.6855, -67.3721) (-69.6086, -67.3228) (-69.5316, -67.2738) (-69.4544, -67.2251) (-69.3772, -67.1768) (-69.2998, -67.1287) (-69.2223, -67.081) (-69.1447, -67.0335) (-69.067, -66.9864) (-68.9892, -66.9396) (-68.9112, -66.8932) (-68.8331, -66.847) (-68.755, -66.8012) (-68.6767, -66.7557) (-68.5982, -66.7106) (-68.5197, -66.6658) (-68.4411, -66.6214) (-68.3623, -66.5773) (-68.2834, -66.5335) (-68.2044, -66.4901) (-68.1253, -66.4471) (-68.046, -66.4044) (-67.9667, -66.3621) (-67.8872, -66.3202) (-67.8076, -66.2786) (-67.7279, -66.2375) (-67.648, -66.1967) (-67.568, -66.1563) (-67.4945, -66.1196) (-67.4369, -66.0912) (-67.3952, -66.0708) (-67.3697, -66.0583) (-67.3602, -66.0537) knots -1 -1 -1 -1 -1 -1 -0.985714 -0.971429 -0.957143 -0.942857 -0.928571 -0.914286 -0.9 -0.885714 -0.871429 -0.857143 -0.842857 -0.828571 -0.814286 -0.8 -0.785714 -0.771429 -0.757143 -0.742857 -0.728571 -0.714286 -0.7 -0.685714 -0.671429 -0.657143 -0.642857 -0.628571 -0.614286 -0.6 -0.585714 -0.571429 -0.557143 -0.542857 -0.528571 -0.514286 -0.5 -0.485714 -0.471429 -0.457143 -0.442857 -0.428571 -0.414286 -0.405839 -0.405839 -0.405839 -0.405839 -0.405839 -0.405839
  arc A172 (-67.5942, -64.7565) -> (-67.3602, -66.0537) centre (2.0032, -52.8695) ccw
  spline S173 degree 5 poles (-67.5942, -64.7565) (-67.6047, -64.7555) (-67.633, -64.7528) (-67.6792, -64.7482) (-67.7431, -64.7417) (-67.8248, -64.733) (-67.9139, -64.7231) (-68.0029, -64.7128) (-68.092, -64.7021) (-68.1811, -64.691) (-68.2702, -64.6795) (-68.3594, -64.6676) (-68.4485, -64.6554) (-68.5377, -64.6427) (-68.6269, -64.6296) (-68.7161, -64.6162) (-68.8053, -64.6024) (-68.8945, -64.5883) (-68.9838, -64.5737) (-69.073, -64.5588) (-69.1623, -64.5436) (-69.2515, -64.528) (-69.3408, -64.512) (-69.4301, -64.4958) (-69.5194, -64.4791) (-69.6086, -64.4621) (-69.6979, -64.4448) (-69.7872, -64.4271) (-69.8765, -64.4092) (-69.9658, -64.3908) (-70.0551, -64.3722) (-70.1444, -64.3532) (-70.2337, -64.3339) (-70.323, -64.3143) (-70.4123, -64.2943) (-70.5016, -64.2741) (-70.5908, -64.2535) (-70.6801, -64.2326) (-70.7694, -64.2114) (-70.8587, -64.1899) (-70.9479, -64.1681) (-71.0372, -64.146) (-71.1264, -64.1236) (-71.1978, -64.1054) (-71.2514, -64.0917) (-71.2871, -64.0824) (-71.3049, -64.0778) knots 0.405839 0.405839 0.405839 0.405839 0.405839 0.405839 0.414286 0.428571 0.442857 0.457143 0.471429 0.485714 0.5 0.514286 0.528571 0.542857 0.557143 0.571429 0.585714 0.6 0.614286 0.628571 0.642857 0.657143 0.671429 0.685714 0.7 0.714286 0.728571 0.742857 0.757143 0.771429 0.785714 0.8 0.814286 0.828571 0.842857 0.857143 0.871429 0.885714 0.9 0.914286 0.928571 0.942857 0.957143 0.971429 0.985714 1 1 1 1 1 1
  arc A173 (-71.4932, -62.7685) -> (-71.3049, -64.0778) centre (2.0032, -52.8695) ccw
  spline S174 degree 5 poles (-71.4932, -62.7685) (-71.4773, -62.759) (-71.4457, -62.7401) (-71.3982, -62.7118) (-71.3348, -62.6742) (-71.2555, -62.6276) (-71.1761, -62.5812) (-71.0966, -62.5351) (-71.017, -62.4894) (-70.9373, -62.4439) (-70.8575, -62.3987) (-70.7776, -62.3538) (-70.6977, -62.3092) (-70.6176, -62.2649) (-70.5375, -62.2209) (-70.4572, -62.1773) (-70.3769, -62.1339) (-70.2965, -62.0908) (-70.216, -62.0481) (-70.1354, -62.0057) (-70.0547, -61.9636) (-69.9739, -61.9218) (-69.893, -61.8804) (-69.812, -61.8392) (-69.731, -61.7985) (-69.6498, -61.758) (-69.5686, -61.7179) (-69.4872, -61.6781) (-69.4058, -61.6387) (-69.3242, -61.5996) (-69.2426, -61.5609) (-69.1609, -61.5225) (-69.0791, -61.4845) (-68.9972, -61.4469) (-68.9152, -61.4096) (-68.8331, -61.3727) (-68.7509, -61.3361) (-68.6687, -61.3) (-68.5863, -61.2642) (-68.5038, -61.2289) (-68.4213, -61.1939) (-68.3386, -61.1593) (-68.2627, -61.128) (-68.2032, -61.1037) (-68.1602, -61.0863) (-68.1338, -61.0757) (-68.124, -61.0718) knots -1 -1 -1 -1 -1 -1 -0.985714 -0.971429 -0.957143 -0.942857 -0.928571 -0.914286 -0.9 -0.885714 -0.871429 -0.857143 -0.842857 -0.828571 -0.814286 -0.8 -0.785714 -0.771429 -0.757143 -0.742857 -0.728571 -0.714286 -0.7 -0.685714 -0.671429 -0.657143 -0.642857 -0.628571 -0.614286 -0.6 -0.585714 -0.571429 -0.557143 -0.542857 -0.528571 -0.514286 -0.5 -0.485714 -0.471429 -0.457143 -0.442857 -0.428571 -0.414286 -0.405839 -0.405839 -0.405839 -0.405839 -0.405839 -0.405839
  arc A174 (-68.2649, -59.7612) -> (-68.124, -61.0718) centre (2.0032, -52.8695) ccw
  spline S175 degree 5 poles (-68.2649, -59.7612) (-68.2753, -59.7595) (-68.3034, -59.7547) (-68.349, -59.7469) (-68.4123, -59.7358) (-68.4932, -59.7213) (-68.5814, -59.7051) (-68.6695, -59.6885) (-68.7576, -59.6715) (-68.8456, -59.654) (-68.9337, -59.6362) (-69.0218, -59.618) (-69.1098, -59.5994) (-69.1979, -59.5804) (-69.2859, -59.561) (-69.3739, -59.5412) (-69.4619, -59.5211) (-69.5499, -59.5006) (-69.6379, -59.4798) (-69.7258, -59.4585) (-69.8138, -59.437) (-69.9017, -59.415) (-69.9896, -59.3928) (-70.0775, -59.3701) (-70.1653, -59.3472) (-70.2532, -59.3239) (-70.341, -59.3002) (-70.4288, -59.2762) (-70.5166, -59.2519) (-70.6044, -59.2273) (-70.6921, -59.2023) (-70.7798, -59.177) (-70.8675, -59.1514) (-70.9552, -59.1254) (-71.0428, -59.0992) (-71.1304, -59.0726) (-71.218, -59.0457) (-71.3056, -59.0185) (-71.3931, -58.991) (-71.4806, -58.9632) (-71.5681, -58.9351) (-71.6555, -58.9066) (-71.743, -58.8779) (-71.8129, -58.8547) (-71.8653, -58.8371) (-71.9002, -58.8254) (-71.9177, -58.8195) knots 0.405839 0.405839 0.405839 0.405839 0.405839 0.405839 0.414286 0.428571 0.442857 0.457143 0.471429 0.485714 0.5 0.514286 0.528571 0.542857 0.557143 0.571429 0.585714 0.6 0.614286 0.628571 0.642857 0.657143 0.671429 0.685714 0.7 0.714286 0.728571 0.742857 0.757143 0.771429 0.785714 0.8 0.814286 0.828571 0.842857 0.857143 0.871429 0.885714 0.9 0.914286 0.928571 0.942857 0.957143 0.971429 0.985714 1 1 1 1 1 1
  arc A175 (-72.0121, -57.5001) -> (-71.9177, -58.8195) centre (2.0032, -52.8695) ccw
  circle A176 centre (2.0032, -52.8695) radius 85
  line L0 (67.0032, 32.1305) -> (-62.9968, 32.1305)
  line L1 (-82.9968, 12.1305) -> (-82.9968, -117.8695)
  line L2 (-62.9968, -137.8695) -> (67.0032, -137.8695)
  line L3 (87.0032, -117.8695) -> (87.0032, 12.1305)
  line L4 (87.0032, 32.1305) -> (-82.9968, -137.8695) construction
  line L5 (-82.9968, 32.1305) -> (87.0032, -137.8695) construction
  circle A177 centre (2.0032, -52.8695) radius 20
  arc A178 (-62.9968, 32.1305) -> (-82.9968, 12.1305) centre (-62.9968, 12.1305) ccw
  arc A179 (87.0032, 12.1305) -> (67.0032, 32.1305) centre (67.0032, 12.1305) ccw
  arc A180 (67.0032, -137.8695) -> (87.0032, -117.8695) centre (67.0032, -117.8695) ccw
  arc A181 (-82.9968, -117.8695) -> (-62.9968, -137.8695) centre (-62.9968, -117.8695) ccw
  circle A182 centre (-66.4862, 15.6199) radius 6
  circle A183 centre (70.4926, 15.6199) radius 6
  circle A184 centre (74.325, -125.1912) radius 6
  point P0 (2.0032, -52.8695)
  dimension "d137" = 170
  dimension "d138" = 170
  dimension "d139" = 40
  dimension "d140" = 20
  dimension "d141" = 12
  dimension "d142" = 12
  dimension "d143" = 12
  constraint horizontal L0
  constraint perpendicular L0 L1
  constraint parallel L0 L2
  constraint parallel L1 L3
  constraint coincident L4 P0
  constraint coincident L5 P0
  constraint coincident P0 A0.centre
  constraint coincident L5.start L0
  constraint coincident L5.start L1
  constraint tangent L0 A178
  constraint tangent L1 A178
  constraint coincident L4.start L0
  constraint coincident L4.start L3
  constraint tangent L0 A179
  constraint tangent L3 A179
  constraint equal A178 A179
  constraint coincident L5.end L3
  constraint coincident L5.end L2
  constraint tangent L3 A180
  constraint tangent L2 A180
  constraint equal A178 A180
  constraint coincident L4.end L2
  constraint coincident L4.end L1
  constraint tangent L2 A181
  constraint tangent L1 A181
  constraint equal A178 A181
  constraint coincident L5 A182.centre
  constraint coincident L4 A183.centre
  constraint coincident L5 A184.centre
  measures "d137" distance of L4.end L5.end
  measures "d138" distance of L5.start L4.end
  measures "d139" diameter of A177
  measures "d140" radius of A178
  measures "d141" diameter of A182
  measures "d142" diameter of A183
  measures "d143" diameter of A184
extrude "Extrude2'''''" add sketch "Sketch2 (2)" along normal blind 15 contours S0 A0 S1 A1 S2 A2 S3 A3 S4 A4 S5 A5 S6 A6 S7 A7 S8 A8 S9 A9 S10 A10 S11 A11 S12 A12 S13 A13 S14 A14 S15 A15 S16 A16 S17 A17 S18 A18 S19 A19 S20 A20 S21 A21 S22 A22 S23 A23 S24 A24 S25 A25 S26 A26 S27 A27 S28 A28 S29 A29 S30 A30 S31 A31 S32 A32 S33 A33 S34 A34 S35 A35 S36 A36 S37 A37 S38 A38 S39 A39 S40 A40 S41 A41 S42 A42 S43 A43 S44 A44 S45 A45 S46 A46 S47 A47 S48 A48 S49 A49 S50 A50 S51 A51 S52 A52 S53 A53 S54 A54 S55 A55 S56 A56 S57 A57 S58 A58 S59 A59 S60 A60 S61 A61 S62 A62 S63 A63 S64 A64 S65 A65 S66 A66 S67 A67 S68 A68 S69 A69 S70 A70 S71 A71 S72 A72 S73 A73 S74 A74 S75 A75 S76 A76 S77 A77 S78 A78 S79 A79 S80 A80 S81 A81 S82 A82 S83 A83 S84 A84 S85 A85 S86 A86 S87 A87 S88 A88 S89 A89 S90 A90 S91 A91 S92 A92 S93 A93 S94 A94 S95 A95 S96 A96 S97 A97 S98 A98 S99 A99 S100 A100 S101 A101 S102 A102 S103 A103 S104 A104 S105 A105 S106 A106 S107 A107 S108 A108 S109 A109 S110 A110 S111 A111 S112 A112 S113 A113 S114 A114 S115 A115 S116 A116 S117 A117 S118 A118 S119 A119 S120 A120 S121 A121 S122 A122 S123 A123 S124 A124 S125 A125 S126 A126 S127 A127 S128 A128 S129 A129 S130 A130 S131 A131 S132 A132 S133 A133 S134 A134 S135 A135 S136 A136 S137 A137 S138 A138 S139 A139 S140 A140 S141 A141 S142 A142 S143 A143 S144 A144 S145 A145 S146 A146 S147 A147 S148 A148 S149 A149 S150 A150 S151 A151 S152 A152 S153 A153 S154 A154 S155 A155 S156 A156 S157 A157 S158 A158 S159 A159 S160 A160 S161 A161 S162 A162 S163 A163 S164 A164 S165 A165 S166 A166 S167 A167 S168 A168 S169 A169 S170 A170 S171 A171 S172 A172 S173 A173 S174 A174 S175 A175 | A176 | A176 L2 L3 A180 | A176 L0 L3 A179 | A176 L0 L1 A178 | A176 L1 L2 A181 bodies 11 in component "Base2"
move_body "Move1" bodies 11 to x (0.999657, 0, 0.026177) y (0, 1, 0) z (-0.026177, 0, 0.999657) at (-95.7786, 0, 2.5322) in component "Base2"
component "Component" placed x (1, 0, 0) y (0, 1, 0) z (0, 0, 1) at (0, 0, 0)
component "planet gear holder" placed x (-0.866544, 0, -0.499101) y (0, 1, 0) z (0.499101, 0, -0.866544) at (0, 25, 0)
component "Component'" placed x (1, 0, 0) y (0, 1, 0) z (0, 0, 1) at (0, -425, 0)
component "SUN  gear" placed x (1, 0, 0) y (0, 1, 0) z (0, 0, 1) at (0, 0, 0)
component "Spur Gear 88 teeth" placed x (1, 0, 0) y (0, 0, 1) z (0, -1, 0) at (-92.8046, -89.257, -204.6171)